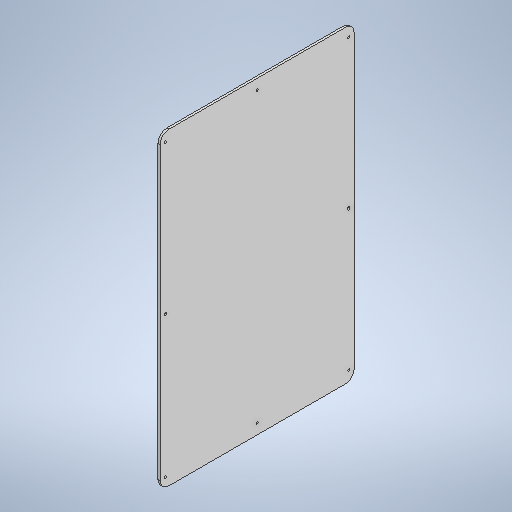
# Autodesk Inventor part: Solar_Panel
Saved by Autodesk Inventor 2025 (Build 290162010, 162A)
## iProperties
Created: 2024-07-15
Part Number: Solar_Panel
Material: Generic
Document SubType Name: Modeling
Designer: vncnt
Density: 1 g/cm^3
Appearance: Default
Author: vncnt
Autodesk Inventor part; units mm, degrees
ref_plane "YZ Plane" through (0, 0, 0) normal (1, 0, 0) x (0, 1, 0)
ref_plane "XZ Plane" through (0, 0, 0) normal (0, 1, 0) x (-1, 0, 0)
ref_plane "XY Plane" through (0, 0, 0) normal (0, 0, 1) x (1, 0, 0)
sketch "Sketch1" plane through (0, 0, 0) normal (1, 0, 0) x (0, 1, 0)
  line L0 (218, -137) -> (-218, -137)
  line L1 (-218, -137) -> (-218, 137)
  line L2 (-218, 137) -> (218, 137)
  line L3 (218, 137) -> (218, -137)
  circle A0 centre (203.4155, 0) radius 1.5
  circle A1 centre (204.9155, 129.5) radius 1.5
  circle A2 centre (203.4155, -129.5) radius 1.5
  arc A3 (-6.1045, 130.9526) -> (-6.1045, 127.9526) centre (-6.1045, 129.4526) ccw
  line L4 (-4.8345, 130.9526) -> (-6.1045, 130.9526)
  line L5 (-6.1045, 127.9526) -> (-4.8345, 127.9526)
  line L6 (-1.8541, 130.9526) -> (-7.8149, 127.9526) construction
  line L7 (-7.8149, 130.9526) -> (-1.8541, 127.9526) construction
  arc A4 (-4.8345, 127.9526) -> (-4.8345, 130.9526) centre (-4.8345, 129.4526) ccw
  line L8 (0, 27.4508) -> (0, -43.9323)
  line L9 (0, 0) -> (50.715, 0)
  circle A5 centre (-203.4155, 0) radius 1.5
  circle A6 centre (-204.9155, 129.5) radius 1.5
  circle A7 centre (-203.4155, -129.5) radius 1.5
  arc A8 (-6.1045, -127.9526) -> (-6.1045, -130.9526) centre (-6.1045, -129.4526) ccw
  line L10 (-4.8345, -130.9526) -> (-6.1045, -130.9526)
  line L11 (-6.1045, -127.9526) -> (-4.8345, -127.9526)
  arc A9 (-4.8345, -130.9526) -> (-4.8345, -127.9526) centre (-4.8345, -129.4526) ccw
  point P0 (218, 0)
  point P1 (-7.8149, -127.9526)
  point P2 (-7.8149, -130.9526)
  dimension "d0" = 436
  dimension "d1" = 274
  dimension "d3" = 3
  dimension "d4" = 3
  dimension "d5" = 3
  dimension "d6" = 259
  dimension "d7" = 129.5
  dimension "d8" = 0
  dimension "d10" = 209.75
  dimension "d11" = 1.27
  dimension "d12" = 3
  dimension "d13" = 3
  dimension "d14" = 1.5
  constraints: 24 end point, 11 symmetric about line, 10 centre point, 8 point on circle, 3 horizontal, 3 midpoint, 3 parallel, 1 perpendicular, 1 point on line, 1 vertical, 5 other
  measures "d0" distance of L1.end L2.end
  measures "d1" distance of L2.end L0.start
  measures "d3" diameter of A0
  measures "d4" diameter of A2
  measures "d5" diameter of A1
  measures "d6" vertical distance of A2.centre A1.centre
  measures "d7" vertical distance of A1.centre A0.centre
  measures "d8" vertical distance of point (218, 0) A0.centre
  measures "d10" distance of A4.centre A1.centre
  measures "d11" distance of A3.centre A4.centre
  measures "d12" diameter of A3
  measures "d13" distance between parallel lines of L4 L5
  measures "d14" distance from line of L5 A3.centre
extrude "Extrusion1" add sketch "Sketch1" along normal blind 3.1
fillet "Fillet1" radius 12.7 4 edges at (1.55, 218, 137) (1.55, 218, -137) (1.55, -218, -137) (1.55, -218, 137)
body "Solid1"
